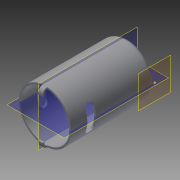
# Autodesk Inventor part: Haz
Saved by Autodesk Inventor 2015 (Build 190159000, 159)
## iProperties
Created: 2014-08-26
Part Number: Haz
Material: Generic
Document SubType Name: Modeling
Designer: laca
Density: 1 g/cm^3
Appearance: Default
Mass: 7.98806 g
Surface Area: 140.627 cm^2
Volume: 7.98806 cm^3
Author: laca
Autodesk Inventor part; units mm, degrees
ref_plane "YZ Plane" through (0, 0, 0) normal (1, 0, 0) x (0, 1, 0)
ref_plane "XZ Plane" through (0, 0, 0) normal (0, 1, 0) x (-1, 0, 0)
ref_plane "XY Plane" through (0, 0, 0) normal (0, 0, 1) x (1, 0, 0)
sketch "Sketch2" plane through (0, 0, 0) normal (0, 1, 0) x (-1, 0, 0)
  line L0 (29.7815, 11.1867) -> (29.7815, -45.8133)
  line L1 (29.7815, -45.8133) -> (11.8815, -45.8133)
  line L2 (29.7815, 11.1867) -> (28.5815, 11.1867)
  line L3 (28.5815, 11.1867) -> (28.5815, -44.6133)
  line L4 (28.5815, -44.6133) -> (12.6405, -44.6133)
  line L5 (12.6405, -44.6133) -> (11.8815, -44.6133)
  line L6 (11.8815, -44.6133) -> (11.8815, -45.8133)
  point P0 (0, 0)
  dimension "d5" = 57
  dimension "d6" = 17.9
  dimension "d7" = 1.2
  dimension "d8" = 1.2
  constraints: 14 end point, 4 perpendicular, 1 horizontal, 1 point on line, 1 vertical
  measures "d5" distance of L0.start L0.end
  measures "d6" distance of L0.end L1.end
  measures "d7" distance between parallel lines of L3 L0
  measures "d8" distance of L5.end L1.end
revolve "Revolution1" add sketch "Sketch2" angle 360 about axis through (-11.8815, 0, -44.6133) along (0, 0, -1)
fillet "Fillet1" radius 3 1 edges at (6.0185, 0, -45.8133)
sketch "Sketch3" plane through (-11.8815, 0, -45.8133) normal (0, 0, -1) x (-1, 0, 0)
  circle A0 centre (0, 0) radius 6.5
  circle A1 centre (0, 0) radius 6
  circle A2 centre (0, 0) radius 12.5
  circle A3 centre (0, 12.5) radius 1.9
  circle A4 centre (0, -12.5) radius 1.9
  line L0 (0, 0) -> (-21.7112, 0)
  point P0 (-11.8815, 0)
  dimension "d17" = 25
  dimension "d11" = 13
  dimension "d12" = 12
  dimension "d18" = 3.8
  dimension "d21" = 360
  constraints: 4 centre point, 2 coincident, 2 end point, 1 horizontal, 1 vertical alignment, 7 other
  measures "d11" diameter of A0
  measures "d12" diameter of A1
  measures "d18" diameter of A3
extrude "Extrusion1" add sketch "Sketch3" along normal blind 4.5 contours A0
extrude "Extrusion2" cut sketch "Sketch3" against normal blind 4.5 contours A1
extrude "Extrusion3" cut sketch "Sketch3" against normal blind 4.5 contours A3 A2 | A2 A3 | A4 A2 | A2 A4
ref_plane "Work Plane1" through (6.0185, 0, -45.8133) normal (1, 0, 0) x (0, 1, 0)
sketch "Sketch4" plane through (6.0185, 0, -45.8133) normal (1, 0, 0) x (0, 1, 0)
  arc A0 (6, 40) -> (6, 46) centre (6, 43) ccw
  line L0 (0, 50.1877) -> (0, 37.5166)
  line L1 (6, 46) -> (0, 46)
  line L2 (6, 40) -> (0, 40)
  arc A1 (-6, 46) -> (-6, 40) centre (-6, 43) ccw
  line L3 (-6, 46) -> (0, 46)
  line L4 (-6, 40) -> (0, 40)
  line L5 (0, 40) -> (0, 0)
  line L6 (14.9, 0) -> (-14.9, 0) projected
  point P0 (0, 45.8133)
  dimension "d25" = 6
  dimension "d27" = 6
  dimension "d29" = 40
  constraints: 12 end point, 4 point on circle, 3 symmetric about line, 2 centre point, 2 perpendicular, 2 point on line, 1 midpoint, 1 tangent, 1 vertical, 1 other
  measures "d25" diameter of A0
  measures "d27" distance from line of L0 A0.centre
  measures "d29" distance of L2.end L5.end
extrude "Extrusion4" cut sketch "Sketch4" against normal through all
sketch "Sketch5" plane through (-11.8815, 0, 11.1867) normal (0, 0, 1) x (1, 0, 0)
  circle A0 centre (0, 0) radius 16.7 projected
  line L0 (-1.5, 17.837) -> (-1.5, 16.6325)
  line L1 (1.5, 17.837) -> (1.5, 16.6325)
  arc A1 (1.5, 17.837) -> (-1.5, 17.837) centre (0, 0) ccw
  arc A2 (1.5, 16.6325) -> (-1.5, 16.6325) centre (0, 0) ccw
  point P0 (11.8815, 0)
  point P1 (1.5, 15.8007)
  constraints: 4 end point, 4 point on circle, 2 centre point, 2 coincident, 1 concentric, 1 vertical
ref_plane "Work Plane2" through (-13.3815, 17.837, 11.1867) normal (-1, 0, 0) x (0, -1, 0)
sketch "Sketch6" plane through (-13.3815, 17.837, 11.1867) normal (-1, 0, 0) x (0, -1, 0)
  line L0 (1.1971, 0) -> (1.1971, 0)
  line L1 (3.1971, 2) -> (4.1971, 2)
  arc A0 (3.1971, 2) -> (1.1971, 0) centre (3.1971, 0) ccw
  point P0 (17.837, -11.1867)
  point P1 (1.1971, 2)
  dimension "d37" = 2
  dimension "d38" = 3
  dimension "d39" = 2
  constraints: 4 end point, 2 point on circle, 2 point on line, 2 tangent, 1 centre point, 1 perpendicular, 1 vertical
  measures "d37" distance of L0.start point (1.197, 2)
  measures "d38" distance of point (1.197, 2) L1.end
  measures "d39" radius of A0
sweep "Sweep1" add profiles "Sketch5" path "Sketch6" path curves A0 L1 contours A0 L0 A1 L1
ref_plane "Work Plane4" through (-11.8815, 0, 11.1867) normal (0, -1, 0) x (1, 0, 0)
mirror "Mirror1" about plane through (-11.8815, 0, 11.1867) normal (0, -1, 0) of "Sweep1"
body "Solid1"
